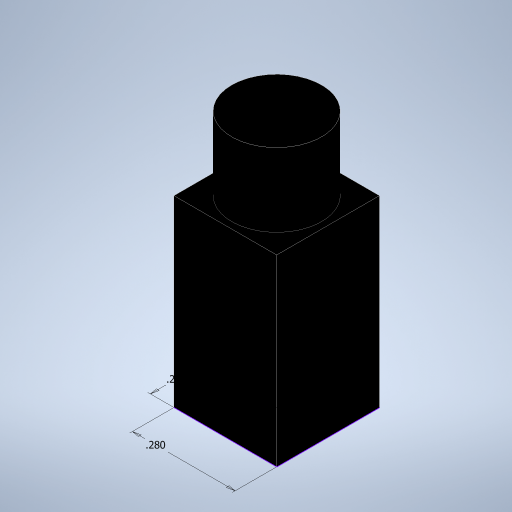
# Autodesk Inventor part: button
Saved by Autodesk Inventor 2023 (Build 270158000, 158)
## iProperties
Created: 2022-11-17
Part Number: button
Material: Generic
Document SubType Name: Modeling
Designer: spfow
Density: 1 g/cm^3
Appearance: Black
Author: spfow
Autodesk Inventor part; units mm, degrees
ref_plane "YZ Plane" through (0, 0, 0) normal (1, 0, 0) x (0, 1, 0)
ref_plane "XZ Plane" through (0, 0, 0) normal (0, 1, 0) x (-1, 0, 0)
ref_plane "XY Plane" through (0, 0, 0) normal (0, 0, 1) x (1, 0, 0)
sketch "Sketch1" plane through (0, 0, 0) normal (0, 1, 0) x (-1, 0, 0)
  circle A0 centre (0, 0) radius 3.1115
  line L0 (3.556, 0) -> (3.556, -3.556)
  line L1 (3.556, -3.556) -> (0, -3.556)
  line L2 (3.556, -3.556) -> (-3.556, -3.556)
  line L3 (-3.556, -3.556) -> (-3.556, 3.556)
  line L4 (-3.556, 3.556) -> (3.556, 3.556)
  line L5 (3.556, 3.556) -> (3.556, -3.556)
  dimension "d0" = 6.223
  dimension "d1" = 3.556
  dimension "d2" = 3.556
  dimension "d3" = 7.112
  dimension "d4" = 7.112
  constraints: 12 end point, 2 parallel, 1 centre point, 1 coincident, 1 horizontal, 1 perpendicular
  measures "d0" diameter of A0
  measures "d1" distance of L0.start L0.end
  measures "d2" distance of L0.end L1.end
  measures "d3" distance of L3.end L4.end
  measures "d4" distance of L4.end L0.end
extrude "Extrusion1" add sketch "Sketch1" along normal blind 17.78 contours A0
extrude "Extrusion2" add sketch "Sketch1" along normal blind 12.7
body "Solid1"
